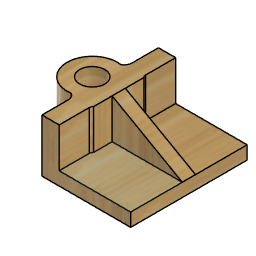
Exercise 4 (Autodesk Fusion 360 design; units mm, degrees)
Autodesk Fusion 360 part; units mm, degrees
sketch "Sketch1" plane through (0, 0, 0) normal (0, 1, 0) x (1, 0, 0)
  line L0 (0, 0) -> (67, 0)
  line L1 (67, 0) -> (67, -10)
  line L2 (67, -10) -> (13, -10)
  line L3 (0, -10) -> (0, 0)
  line L4 (0, 0) -> (13, 0)
  line L5 (13, -10) -> (13, -40)
  line L6 (13, -40) -> (0, -40)
  line L7 (0, -40) -> (0, 0)
  dimension "d1" = 67
  dimension "d2" = 10
  dimension "d3" = 13
  dimension "d4" = 40
  constraint horizontal L0
  constraint vertical L1
  constraint horizontal L2
  constraint vertical L3
  constraint coincident L0.start L3.end
  constraint horizontal L4
  constraint vertical L5
  constraint horizontal L6
  constraint vertical L7
  measures "d1" distance of L0.start L0.end
  measures "d2" distance of L0.start L3.start
  measures "d3" distance of L0.start L4.end
  measures "d4" distance of L0.start L6.end
extrude "Extrude1" add sketch "Sketch1" along normal blind 88
sketch "Sketch2" plane through (0, 0, 40) normal (0, 0, 1) x (-1, 0, 0)
  line L0 (0, 0) -> (-13, 0)
  line L1 (-13, 0) -> (-13, -88)
  line L2 (-13, -88) -> (0, -88)
  line L3 (0, -88) -> (0, 0)
  line L4 (-13, 0) -> (-13, -44) construction
  arc A0 (3.0968, -62.7769) -> (3.0968, -25.2231) centre (6, -44) ccw
  line L5 (0, -68.0278) -> (0, -95) construction
  arc A1 (3.0968, -62.7769) -> (0, -68.0278) centre (6, -68.0278) ccw
  line L6 (0, -19.9722) -> (0, 0) construction
  arc A2 (0, -19.9722) -> (3.0968, -25.2231) centre (6, -19.9722) ccw
  dimension "d11" = 6
  dimension "d12" = 6
  constraint coincident L0.end L1.start
  constraint perpendicular L0 L4
  constraint perpendicular L2 L5
  constraint tangent L5 A1
  constraint coincident L0.start L3.end
  constraint tangent L6 A2
  measures "d11" radius of A1
  measures "d12" radius of A2
extrude "Extrude2" add sketch "Sketch2" against normal blind 40 contours L3 A0 A1 A2
sketch "Sketch3" plane through (0, 0, 40) normal (0, 0, 1) x (-1, 0, 0)
  line L0 (0, 0) -> (-13, 0)
  line L1 (-13, 0) -> (-13, -88)
  line L2 (-13, -88) -> (0, -88)
  line L3 (0, -88) -> (0, -68.0278)
  arc A0 (3.0968, -62.7769) -> (0, -68.0278) centre (6, -68.0278) ccw
  arc A1 (3.0968, -62.7769) -> (3.0968, -25.2231) centre (6, -44) ccw
  arc A2 (0, -19.9722) -> (3.0968, -25.2231) centre (6, -19.9722) ccw
  line L4 (0, -19.9722) -> (0, 0)
  line L5 (6, -44) -> (-13, -44) construction
  constraint coincident A1.centre L5.start
  constraint midpoint L1 L5.end
hole "Hole1" at (-6, 44, 40) direction (0, 0, -1) diameter 19 depth 50 tip angle 118
sketch "Sketch4" plane through (0, 0, 40) normal (0, 0, 1) x (-1, 0, 0)
  circle A0 centre (6, -44) radius 9.5
  line L0 (0, 0) -> (-13, 0)
  line L1 (-13, 0) -> (-13, -88)
  line L2 (-13, -88) -> (0, -88)
  line L3 (0, -88) -> (0, -68.0278)
  arc A1 (3.0968, -62.7769) -> (0, -68.0278) centre (6, -68.0278) ccw
  arc A2 (3.0968, -62.7769) -> (3.0968, -25.2231) centre (6, -44) ccw
  arc A3 (0, -19.9722) -> (3.0968, -25.2231) centre (6, -19.9722) ccw
  line L4 (0, -19.9722) -> (0, 0)
  line L5 (-14, -63) -> (-14, -25)
  line L6 (-13, -25) -> (-14, -25)
  line L7 (-13, -63) -> (-14, -63)
  dimension "d19" = 25
  constraint perpendicular L5 L6
  constraint perpendicular L5 L7
  measures "d19" distance of L0.end L6.start
extrude "Extrude3" add sketch "Sketch4" against normal blind 30 contours L1 L5 L6 L7
fillet "Fillet1" radius 3 1 edges at (13, 25, 25)
fillet "Fillet2" radius 3 1 edges at (13, 63, 25)
ref_plane "WorkPlane1" through (0, 44, 0) normal (0, 1, 0) x (0, 0, 1)
sketch "Sketch5" plane through (0, 44, 0) normal (0, 1, 0) x (1, 0, 0)
  line L0 (14, -40) -> (67, -10)
rib "Rib1" add thickness 10 on both sides direction (-0.492598, 0, -0.870257) up to next extending the curves path "Sketch5" along L0
sketch "Sketch6" plane through (0, 0, 10) normal (0, 0, 1) x (-1, 0, 0)
  line L0 (-67, -39) -> (-14, -39)
  line L1 (-14, -39) -> (-14, -25)
  arc A0 (-14, -25) -> (-13, -22.7639) centre (-16, -22.7639) ccw
  line L2 (-13, -22.7639) -> (-13, 0)
  line L3 (-13, 0) -> (-67, 0)
  line L4 (-67, 0) -> (-67, -39)
